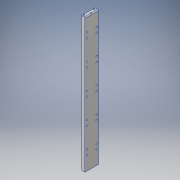
# Autodesk Inventor part: Winch_Plate_Front
Saved by Autodesk Inventor 2016 (Build 200138000, 138)
## iProperties
Created: 2016-05-06
Part Number: Winch_Plate_Front
Material: Aluminum 6061
Document SubType Name: Modeling
Designer: agmle
Density: 2.7 g/cm^3
Appearance: Aluminum - Flat
Author: agmle
Autodesk Inventor part; units mm, degrees
ref_plane "YZ Plane" through (0, 0, 0) normal (1, 0, 0) x (0, 1, 0)
ref_plane "XZ Plane" through (0, 0, 0) normal (0, 1, 0) x (-1, 0, 0)
ref_plane "XY Plane" through (0, 0, 0) normal (0, 0, 1) x (1, 0, 0)
sketch "Sketch1" plane through (0, 0, 0) normal (0, 1, 0) x (-1, 0, 0)
  line L0 (16.2053, 25.1534) -> (3.5053, 25.1534)
  line L1 (3.5053, 25.1534) -> (3.5053, -25.6466)
  line L2 (3.5053, -25.6466) -> (16.2053, -25.6466)
  line L3 (16.2053, -25.6466) -> (16.2053, 25.1534)
  point P0 (0, 0)
  dimension "d0" = 50.8
  dimension "d1" = 12.7
  constraints: 8 end point, 2 parallel, 1 horizontal, 1 perpendicular
  measures "d0" distance of L2.end L0.start
  measures "d1" distance of L1.end L2.end
extrude "Extrusion1" add sketch "Sketch1" along normal blind 504.952
sketch "Sketch2" plane through (-3.5053, 0, 25.1534) normal (1, 0, 0) x (0, 0, -1)
  line L0 (6.985, 52.451) -> (6.985, 71.501) construction
  line L1 (6.985, 71.501) -> (43.815, 71.501) construction
  line L2 (43.815, 71.501) -> (43.815, 52.451) construction
  line L3 (43.815, 52.451) -> (6.985, 52.451) construction
  line L4 (6.985, 61.976) -> (0, 61.976) construction
  line L5 (0, 0) -> (0, 504.952) construction
  line L6 (43.815, 61.976) -> (50.8, 61.976) construction
  line L7 (50.8, 0) -> (50.8, 504.952) construction
  line L8 (6.985, 147.701) -> (6.985, 166.751) construction
  line L9 (6.985, 157.226) -> (0, 157.226) construction
  line L10 (6.985, 166.751) -> (43.815, 166.751) construction
  line L11 (43.815, 147.701) -> (6.985, 147.701) construction
  line L12 (43.815, 166.751) -> (43.815, 147.701) construction
  line L13 (43.815, 157.226) -> (50.8, 157.226) construction
  line L14 (6.985, 242.951) -> (6.985, 262.001) construction
  line L15 (6.985, 252.476) -> (0, 252.476) construction
  line L16 (6.985, 262.001) -> (43.815, 262.001) construction
  line L17 (43.815, 242.951) -> (6.985, 242.951) construction
  line L18 (43.815, 262.001) -> (43.815, 242.951) construction
  line L19 (43.815, 252.476) -> (50.8, 252.476) construction
  line L20 (6.985, 338.201) -> (6.985, 357.251) construction
  line L21 (6.985, 347.726) -> (0, 347.726) construction
  line L22 (6.985, 357.251) -> (43.815, 357.251) construction
  line L23 (43.815, 338.201) -> (6.985, 338.201) construction
  line L24 (43.815, 357.251) -> (43.815, 338.201) construction
  line L25 (43.815, 347.726) -> (50.8, 347.726) construction
  line L26 (6.985, 433.451) -> (6.985, 452.501) construction
  line L27 (6.985, 442.976) -> (0, 442.976) construction
  line L28 (6.985, 452.501) -> (43.815, 452.501) construction
  line L29 (43.815, 433.451) -> (6.985, 433.451) construction
  line L30 (43.815, 452.501) -> (43.815, 433.451) construction
  line L31 (43.815, 442.976) -> (50.8, 442.976) construction
  point P0 (25.1534, 0)
  dimension "d4" = 36.83
  dimension "d5" = 19.05
  dimension "d6" = 6.985
  dimension "d9" = 95.25
  constraints: 60 end point, 8 point on line, 3 midpoint, 2 equal length, 2 vertical, 1 horizontal, 1 parallel, 1 perpendicular, 56 other
  measures "d4" distance of L2.end L0.start
  measures "d5" distance of L1.end L2.end
  measures "d6" distance of L4.start L4.end
  measures "d9" distance of L0.start L8.start
hole "Hole1" at (-3.5053, 52.451, 18.1684) at (-3.5053, 52.451, -18.6616) at (-3.5053, 71.501, -18.6616) at (-3.5053, 71.501, 18.1684) at (-3.5053, 147.701, 18.1684) at (-3.5053, 166.751, 18.1684) at (-3.5053, 166.751, -18.6616) at (-3.5053, 147.701, -18.6616) at (-3.5053, 242.951, 18.1684) at (-3.5053, 262.001, 18.1684) at (-3.5053, 262.001, -18.6616) at (-3.5053, 242.951, -18.6616) at (-3.5053, 338.201, 18.1684) at (-3.5053, 357.251, 18.1684) at (-3.5053, 357.251, -18.6616) at (-3.5053, 338.201, -18.6616) at (-3.5053, 433.451, 18.1684) at (-3.5053, 452.501, 18.1684) at (-3.5053, 452.501, -18.6616) at (-3.5053, 433.451, -18.6616) direction (-1, 0, 0) diameter 5.1054 end through all clearance for "Socket Head Cap Screw" size "#10" standard "Ansi Unified Screw Threads"
sketch "Sketch3" plane through (0, 0, 0) normal (0, -1, 0) x (1, 0, 0)
  line L0 (-3.5053, 25.1534) -> (-3.5053, -25.6466) construction
  line L1 (-3.5053, -0.2466) -> (-16.2053, -0.2466) construction
  line L2 (-16.2053, -25.6466) -> (-16.2053, 25.1534) construction
  line L3 (-13.0303, 18.8034) -> (-13.0303, -0.2466) construction
  line L4 (-13.0303, -19.2966) -> (-13.0303, -0.2466) construction
  line L5 (-16.2053, 25.1534) -> (-3.5053, 25.1534) construction
  point P0 (0, 0)
  point P1 (-6.6803, -0.2466)
  dimension "d21" = 3.175
  dimension "d22" = 3.175
  dimension "d23" = 6.35
  constraints: 6 end point, 2 collinear, 2 midpoint, 2 point on line, 1 perpendicular
  measures "d21" distance from line of L0 point (-6.68, -0.247)
  measures "d22" distance between parallel lines of L2 L4
  measures "d23" distance from line of L5 L3.start
hole "Hole2" at (-13.0303, 0, 18.8034) at (-6.6803, 0, -0.2466) at (-13.0303, 0, -19.2966) direction (0, 1, 0) diameter 3.9624 depth 19.05 tip angle 118 thread size "10-32 UNF" class "2B" standard "ANSI Unified Screw Threads"
sketch "Sketch4" plane through (0, 504.952, 0) normal (0, 1, 0) x (1, 0, 0)
  circle A0 centre (-6.6803, 0.2466) radius 1.9812 construction
  circle A1 centre (-13.0303, 19.2966) radius 1.9812 construction
  circle A2 centre (-13.0303, -18.8034) radius 1.9812 construction
  point P0 (0, 0)
  dimension "d38" = 6.35
  dimension "d39" = 38.1
  constraints: 3 coincident
  measures "d38" horizontal distance of A1.centre A0.centre
  measures "d39" distance of A2.centre point (-13.03, 19.297)
hole "Hole3" at (-6.6803, 504.952, -0.2466) at (-13.0303, 504.952, -19.2966) at (-13.0303, 504.952, 18.8034) direction (0, -1, 0) diameter 3.9624 depth 19.05 tip angle 118 thread size "10-32 UNF" class "2B" standard "ANSI Unified Screw Threads"
fillet "Fillet1" radius 3.175 2 edges at (-16.2053, 0, -0.2466) (-3.5053, 504.952, -0.2466)
body "Solid1"
